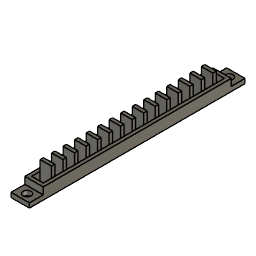
window (Autodesk Fusion 360 design; units mm, degrees)
Autodesk Fusion 360 part; units mm, degrees
sketch "スケッチ1" plane through (0, 0, 0) normal (0, 0, 1) x (1, 0, 0)
  line L0 (1.5, 1.2) -> (3.5, 1.2)
  line L1 (3.5, 1.2) -> (3.5, 2.4)
  line L2 (3.5, 2.4) -> (1.5, 2.4)
  line L3 (1.5, 2.4) -> (1.5, 1.2)
  line L4 (1.5, 6.2) -> (3.5, 6.2)
  line L5 (3.5, 7.4) -> (1.5, 7.4)
  line L6 (3.5, 6.2) -> (3.5, 7.4)
  line L7 (1.5, 7.4) -> (1.5, 6.2)
  line L8 (1.5, 11.2) -> (3.5, 11.2)
  line L9 (3.5, 12.4) -> (1.5, 12.4)
  line L10 (3.5, 11.2) -> (3.5, 12.4)
  line L11 (1.5, 12.4) -> (1.5, 11.2)
  line L12 (1.5, 16.2) -> (3.5, 16.2)
  line L13 (3.5, 17.4) -> (1.5, 17.4)
  line L14 (3.5, 16.2) -> (3.5, 17.4)
  line L15 (1.5, 17.4) -> (1.5, 16.2)
  line L16 (1.5, 21.2) -> (3.5, 21.2)
  line L17 (3.5, 22.4) -> (1.5, 22.4)
  line L18 (3.5, 21.2) -> (3.5, 22.4)
  line L19 (1.5, 22.4) -> (1.5, 21.2)
  line L20 (1.5, 26.2) -> (3.5, 26.2)
  line L21 (3.5, 27.4) -> (1.5, 27.4)
  line L22 (3.5, 26.2) -> (3.5, 27.4)
  line L23 (1.5, 27.4) -> (1.5, 26.2)
  line L24 (1.5, 31.2) -> (3.5, 31.2)
  line L25 (3.5, 32.4) -> (1.5, 32.4)
  line L26 (3.5, 31.2) -> (3.5, 32.4)
  line L27 (1.5, 32.4) -> (1.5, 31.2)
  line L28 (1.5, 36.2) -> (3.5, 36.2)
  line L29 (3.5, 37.4) -> (1.5, 37.4)
  line L30 (3.5, 36.2) -> (3.5, 37.4)
  line L31 (1.5, 37.4) -> (1.5, 36.2)
  line L32 (1.5, 41.2) -> (3.5, 41.2)
  line L33 (3.5, 42.4) -> (1.5, 42.4)
  line L34 (3.5, 41.2) -> (3.5, 42.4)
  line L35 (1.5, 42.4) -> (1.5, 41.2)
  line L36 (1.5, 46.2) -> (3.5, 46.2)
  line L37 (3.5, 47.4) -> (1.5, 47.4)
  line L38 (3.5, 46.2) -> (3.5, 47.4)
  line L39 (1.5, 47.4) -> (1.5, 46.2)
  line L40 (1.5, 51.2) -> (3.5, 51.2)
  line L41 (3.5, 52.4) -> (1.5, 52.4)
  line L42 (3.5, 51.2) -> (3.5, 52.4)
  line L43 (1.5, 52.4) -> (1.5, 51.2)
  line L44 (1.5, 56.2) -> (3.5, 56.2)
  line L45 (3.5, 57.4) -> (1.5, 57.4)
  line L46 (3.5, 56.2) -> (3.5, 57.4)
  line L47 (1.5, 57.4) -> (1.5, 56.2)
  line L48 (1.5, 61.2) -> (3.5, 61.2)
  line L49 (3.5, 62.4) -> (1.5, 62.4)
  line L50 (3.5, 61.2) -> (3.5, 62.4)
  line L51 (1.5, 62.4) -> (1.5, 61.2)
  line L52 (1.5, 66.2) -> (3.5, 66.2)
  line L53 (3.5, 67.4) -> (1.5, 67.4)
  line L54 (3.5, 66.2) -> (3.5, 67.4)
  line L55 (1.5, 67.4) -> (1.5, 66.2)
  line L56 (1.5, 71.2) -> (3.5, 71.2)
  line L57 (3.5, 72.4) -> (1.5, 72.4)
  line L58 (3.5, 71.2) -> (3.5, 72.4)
  line L59 (1.5, 72.4) -> (1.5, 71.2)
  line L60 (1.5, 76.2) -> (3.5, 76.2)
  line L61 (3.5, 77.4) -> (1.5, 77.4)
  line L62 (3.5, 76.2) -> (3.5, 77.4)
  line L63 (1.5, 77.4) -> (1.5, 76.2)
  line L64 (0, 78.6) -> (5, 78.6)
  line L65 (5, 78.6) -> (5, 0)
  line L66 (5, 0) -> (0, 0)
  line L67 (0, 0) -> (0, 78.6)
  line L68 (6.5, -1.5) -> (-1.5, -1.5)
  line L69 (-1.5, -1.5) -> (-1.5, 80.1)
  line L70 (-1.5, 80.1) -> (6.5, 80.1)
  line L71 (6.5, 80.1) -> (6.5, -1.5)
  line L72 (0, 5.1) -> (5, 5.1)
  line L73 (5, 5.1) -> (5, 3.6)
  line L74 (5, 3.6) -> (0, 3.6)
  line L75 (0, 3.6) -> (0, 5.1)
  line L76 (5, 8.6) -> (0, 8.6)
  line L77 (0, 10.1) -> (5, 10.1)
  line L78 (5, 13.6) -> (0, 13.6)
  line L79 (0, 15.1) -> (5, 15.1)
  line L80 (5, 18.6) -> (0, 18.6)
  line L81 (0, 20.1) -> (5, 20.1)
  line L82 (5, 23.6) -> (0, 23.6)
  line L83 (0, 25.1) -> (5, 25.1)
  line L84 (5, 28.6) -> (0, 28.6)
  line L85 (0, 30.1) -> (5, 30.1)
  line L86 (5, 33.6) -> (0, 33.6)
  line L87 (0, 35.1) -> (5, 35.1)
  line L88 (5, 38.6) -> (0, 38.6)
  line L89 (0, 40.1) -> (5, 40.1)
  line L90 (5, 43.6) -> (0, 43.6)
  line L91 (0, 45.1) -> (5, 45.1)
  line L92 (5, 48.6) -> (0, 48.6)
  line L93 (0, 50.1) -> (5, 50.1)
  line L94 (5, 53.6) -> (0, 53.6)
  line L95 (0, 55.1) -> (5, 55.1)
  line L96 (5, 58.6) -> (0, 58.6)
  line L97 (0, 60.1) -> (5, 60.1)
  line L98 (5, 63.6) -> (0, 63.6)
  line L99 (0, 65.1) -> (5, 65.1)
  line L100 (5, 68.6) -> (0, 68.6)
  line L101 (0, 70.1) -> (5, 70.1)
  line L102 (5, 73.6) -> (0, 73.6)
  line L103 (0, 75.1) -> (5, 75.1)
  line L104 (-1.5, 80.1) -> (6.5, 80.1)
  line L105 (6.5, 80.1) -> (6.5, 86.1)
  line L106 (6.5, 86.1) -> (-1.5, 86.1)
  line L107 (-1.5, 86.1) -> (-1.5, 80.1)
  circle A0 centre (2.5, 83.1) radius 1.75
  line L108 (-1.5, -1.5) -> (6.5, -1.5)
  line L109 (6.5, -1.5) -> (6.5, -7.5)
  line L110 (6.5, -7.5) -> (-1.5, -7.5)
  line L111 (-1.5, -7.5) -> (-1.5, -1.5)
  circle A1 centre (2.5, -4.5) radius 1.75
  dimension "d1" = 2
  dimension "d2" = 1.2
  dimension "d5" = 0
  dimension "d6" = 75
  dimension "d7" = 78.6
  dimension "d8" = 1.2
  dimension "d9" = 5
  dimension "d10" = 1.5
  dimension "d11" = -1.5
  dimension "d12" = 1.5
  dimension "d15" = 0
  dimension "d16" = 70
  dimension "d17" = 1.2
  dimension "d18" = 8
  dimension "d19" = 6
  dimension "d20" = 3.5
  dimension "d21" = 4
  dimension "d22" = 3
  dimension "d23" = 8
  dimension "d24" = 6
  dimension "d25" = 3.5
  dimension "d26" = 4
  dimension "d27" = 3
  constraint horizontal L0
  constraint vertical L1
  constraint horizontal L2
  constraint vertical L3
  constraint horizontal L64
  constraint vertical L65
  constraint horizontal L66
  constraint vertical L67
  constraint coincident L66.end L67.start
  constraint horizontal L72
  constraint vertical L73
  constraint horizontal L74
  constraint vertical L75
  constraint coincident L65 L73.end
  constraint coincident L67 L72.start
  constraint horizontal L104
  constraint vertical L105
  constraint horizontal L106
  constraint vertical L107
  constraint horizontal L108
  constraint vertical L109
  constraint horizontal L110
  constraint vertical L111
  measures "d1" distance of L0.start L0.end
  measures "d2" distance of L0.start L2.end
  measures "d7" distance of L64.start L66.end
  measures "d8" distance of L66.end L0
  measures "d9" distance of L65.end L66.end
  measures "d10" distance of L3 L67
  measures "d12" distance of L72 L74
  measures "d17" distance of L2 L74
  measures "d18" distance of L69.end L70.end
  measures "d19" distance of L69.end L106.end
  measures "d20" diameter of A0
  measures "d21" distance of L107 A0.centre
  measures "d22" distance of L106 A0.centre
  measures "d23" distance of L68.end L68.start
  measures "d24" distance of L68.end L110.end
  measures "d25" diameter of A1
  measures "d26" distance of L111 A1.centre
  measures "d27" distance of L110 A1.centre
extrude "押し出し1" add sketch "スケッチ1" along normal blind 5 contours L68 L69 L70 L71 L104 L108
extrude "押し出し2" add sketch "スケッチ1" along normal blind 9.5 contours L65 L67 L102 L103 | L65 L67 L100 L101 | L65 L67 L98 L99 | L65 L67 L96 L97 | L65 L67 L94 L95 | L65 L67 L92 L93 | L65 L67 L90 L91 | L65 L67 L88 L89 | L65 L67 L86 L87 | L65 L67 L84 L85 | L65 L67 L82 L83 | L65 L67 L80 L81 | L65 L67 L78 L79 | L65 L67 L76 L77 | L65 L67 L72 L73 L74 L75
extrude "押し出し3" add sketch "スケッチ1" along normal blind 2 contours L68 L108 L109 L110 L111 | L70 L104 L105 L106 L107
equation "d7 = 80 mm - 1.4 mm"
